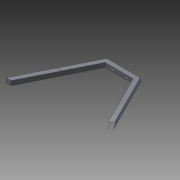
# Autodesk Inventor part: CAVALETE_INFERIOR
Saved by Autodesk Inventor 2015 (Build 190159000, 159)
## iProperties
Manager: Standard
Created: 2016-02-21
Part Number: CAVALETE_INFERIOR
Material: SAE 1010/1020
Document SubType Name: Modeling
Designer: Everton
Authority: Rafael Salvador
Manufacturer: Standard
Standards Organization: Custom
Density: 7.86 g/cm^3
Appearance: Steel
Author: Everton
Comments: -
Revision Number: 00
Autodesk Inventor part; units mm, degrees
ref_plane "YZ Plane" through (0, 0, 0) normal (1, 0, 0) x (0, 1, 0)
ref_plane "XZ Plane" through (0, 0, 0) normal (0, 1, 0) x (-1, 0, 0)
ref_plane "XY Plane" through (0, 0, 0) normal (0, 0, 1) x (1, 0, 0)
sketch "Sketch1" plane through (0, 0, 0) normal (0, 0, 1) x (1, 0, 0)
  line L0 (9.7407, 1114.2593) -> (159.7407, 1114.2593)
  line L1 (9.7407, 1114.2593) -> (-140.2593, 1114.2593)
  line L2 (-290.2593, 814.2593) -> (-140.2593, 1114.2593)
  line L3 (159.7407, 1114.2593) -> (459.7407, 514.2593)
  line L4 (135.0194, 1074.2593) -> (9.7407, 1074.2593)
  line L5 (9.7407, 1074.2593) -> (-115.5379, 1074.2593)
  line L6 (-115.5379, 1074.2593) -> (-245.5379, 814.2593)
  line L7 (9.7407, 1114.2593) -> (159.7407, 1114.2593)
  line L8 (9.7407, 1114.2593) -> (-140.2593, 1114.2593)
  line L9 (-440.2593, 514.2593) -> (-140.2593, 1114.2593)
  line L10 (159.7407, 1114.2593) -> (309.9483, 813.8441)
  line L11 (135.0194, 1074.2593) -> (9.7407, 1074.2593)
  line L12 (9.7407, 1074.2593) -> (-115.5379, 1074.2593)
  line L13 (-115.5379, 1074.2593) -> (-245.5379, 814.2593)
  line L14 (-245.5379, 814.2593) -> (-290.2593, 814.2593)
  line L15 (265.227, 813.8441) -> (309.9483, 813.8441)
  line L16 (265.227, 813.8441) -> (135.0194, 1074.2593)
  line L17 (415.0194, 514.2593) -> (135.0194, 1074.2593)
  line L18 (-395.5379, 514.2593) -> (-440.2593, 514.2593)
  line L19 (-245.5379, 814.2593) -> (-395.5379, 514.2593)
  line L20 (-440.2593, 514.2593) -> (-395.5379, 514.2593)
  line L21 (415.0194, 514.2593) -> (459.7407, 514.2593)
  point P0 (0, 0)
  dimension "d13" = 300
  constraints: 44 end point, 4 horizontal, 2 point on line, 1 midpoint
  measures "d13" distance from line of L6.end L1
extrude "Extrusion1" add sketch "Sketch1" along normal blind 40 contours L0 L3 L15 L16 L4 L5 L6 L14 L2 L1
fillet "Fillet1" radius 0.5 10 edges at (72.3801, 1074.2593, 40) (72.3801, 1074.2593, 0) (200.1232, 944.0517, 40) (234.8445, 964.0517, 40) (-65.2593, 1114.2593, 40) (-215.2593, 964.2593, 40) (-180.5379, 944.2593, 40) (-267.8986, 814.2593, 40) (-180.5379, 944.2593, 0) (234.8445, 964.0517, 0)
fillet "Fillet2" radius 0.5 1 edges at (200.1232, 944.0517, 0)
fillet "Fillet3" radius 0.5 3 edges at (159.7407, 1114.2593, 20) (84.4612, 1114.2593, 0) (-215.2593, 964.2593, 0)
sketch "Sketch2" plane through (-140.2593, 1114.2593, 0.5) normal (0, 1, 0) x (1, 0, 0)
  line L0 (300.1382, -39) -> (300.1382, 0) projected
  line L1 (300.1382, -19.5) -> (0, -19.5)
  line L2 (0, 0) -> (0, -39) projected
  circle A0 centre (150.0691, -19.5) radius 1.5
  point P0 (140.2593, 0.5)
  dimension "d14" = 3
  constraints: 3 midpoint, 2 end point, 1 centre point
  measures "d14" diameter of A0
extrude "Extrusion2" cut sketch "Sketch2" against normal blind 10
extrude "Extrusion3" add sketch "Sketch1" along normal blind 40 contours L3 L21 L17 L15 | L14 L19 L18 L9
sketch "Sketch3" plane through (-140.2593, 1114.2593, 0.5) normal (0, 1, 0) x (1, 0, 0)
  point P0 (140.2593, 0.5)
sketch "Sketch4" plane through (-140.2593, 1114.2593, 0.5) normal (0, 1, 0) x (1, 0, 0)
  circle A0 centre (150.0691, -19.5) radius 1.5 projected
  line L0 (0, 0) -> (299.691, 0) projected
  line L1 (0, 0) -> (0, -39) projected
  line L2 (299.691, -39) -> (0, -39) projected
  line L3 (299.691, 0) -> (299.691, -39) projected
  line L4 (200.1691, -14.5) -> (225.9691, -14.5) projected
  line L5 (225.9691, -24.5) -> (200.1691, -24.5) projected
  arc A1 (225.9691, -24.5) -> (225.9691, -14.5) centre (225.9691, -19.5) ccw projected
  arc A2 (200.1691, -14.5) -> (200.1691, -24.5) centre (200.1691, -19.5) ccw projected
  arc A3 (74.1691, -14.5) -> (74.1691, -24.5) centre (74.1691, -19.5) ccw projected
  line L6 (74.1691, -14.5) -> (99.9691, -14.5) projected
  line L7 (74.1691, -24.5) -> (99.9691, -24.5) projected
  arc A4 (99.9691, -24.5) -> (99.9691, -14.5) centre (99.9691, -19.5) ccw projected
  point P0 (140.2593, 0.5)
extrude "Extrusion4" cut sketch "Sketch4" against normal blind 50 contours L4 A1 L5 A2 | L6 A4 L7 A3
body "Solid1"
